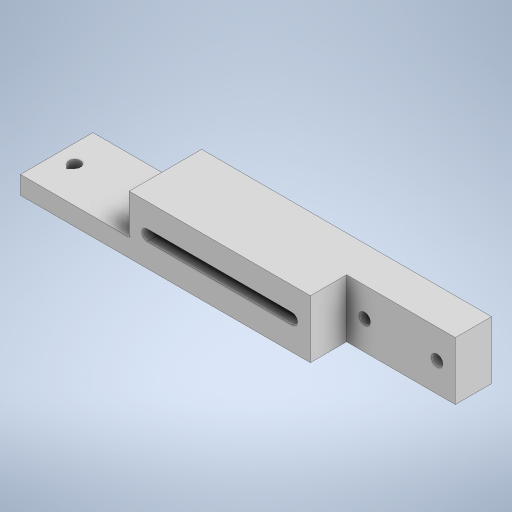
# Autodesk Inventor part: middle_hole
Saved by Autodesk Inventor 2023 (Build 270158000, 158)
## iProperties
Created: 2023-11-20
Part Number: middle_hole
Material: Všeobecné
Document SubType Name: Modeling
Designer: zavrel
Density: 1 g/cm^3
Appearance: Výchozí
Author: zavrel
Autodesk Inventor part; units mm, degrees
ref_plane "YZ Plane" through (0, 0, 0) normal (1, 0, 0) x (0, 1, 0)
ref_plane "XZ Plane" through (0, 0, 0) normal (0, 1, 0) x (-1, 0, 0)
ref_plane "XY Plane" through (0, 0, 0) normal (0, 0, 1) x (1, 0, 0)
sketch "Náčrt1" plane through (0, 0, 0) normal (0, 1, 0) x (-1, 0, 0)
  line L0 (0, 0) -> (110, 0)
  line L1 (110, 0) -> (110, -20)
  line L2 (110, -20) -> (0, -20)
  line L3 (0, -20) -> (0, 0)
  line L4 (55, -20) -> (55, 0) construction
  line L5 (110, -10) -> (0, -10) construction
  circle A0 centre (105, -10) radius 1.6
  circle A1 centre (85, -10) radius 1.6
  line L6 (105, -10) -> (105, -4.8731) construction
  line L7 (85, -10) -> (85, -4.8731) construction
  line L8 (105, -7.7373) -> (103.8686, -8.8686)
  line L9 (105, -7.7373) -> (106.1314, -8.8686)
  line L10 (85, -7.7373) -> (83.8686, -8.8686)
  line L11 (85, -7.7373) -> (86.1314, -8.8686)
  dimension "d0" = 20
  dimension "d1" = 110
  dimension "d4" = 3.2
  dimension "d6" = 25
  dimension "d7" = 5
  dimension "d49" = 90
  dimension "d50" = 90
  constraints: 24 end point, 4 midpoint, 3 point on line, 2 centre point, 2 parallel, 2 point on circle, 2 tangent, 2 vertical, 1 equal radius, 1 horizontal, 1 perpendicular
  measures "d0" distance between parallel lines of L2 L0
  measures "d1" distance of L1.end L2.end
  measures "d4" diameter of A0
  measures "d6" distance from line of L1 L7.start
  measures "d7" distance from line of L1 L6.start
  measures "d49" angle of L9 L8
  measures "d50" angle of L11 L10
extrude "Vysunutí1" add sketch "Náčrt1" along normal blind 16
sketch "Náčrt2" plane through (0, 16, 0) normal (0, 1, 0) x (1, 0, 0)
  line L0 (0, 20) -> (-110, 20) projected
  line L1 (-110, 20) -> (-110, 0) projected
  line L2 (-110, 0) -> (0, 0) projected
  line L3 (0, 0) -> (0, 20) projected
  arc A0 (-83.8686, 8.8686) -> (-86.1314, 8.8686) centre (-85, 10) ccw projected
  arc A1 (-103.8686, 8.8686) -> (-106.1314, 8.8686) centre (-105, 10) ccw projected
  line L4 (-80, 0) -> (-80, 20)
  line L5 (-30, 0) -> (-30, 20)
  arc A2 (-103.8686, 8.8686) -> (-106.1314, 8.8686) centre (-105, 10) ccw construction
  arc A3 (-83.8686, 8.8686) -> (-86.1314, 8.8686) centre (-85, 10) ccw projected
  line L6 (-85, 7.7373) -> (-86.1314, 8.8686) projected
  line L7 (-83.8686, 8.8686) -> (-85, 7.7373) projected
  line L8 (-105, 7.7373) -> (-106.1314, 8.8686) projected
  line L9 (-103.8686, 8.8686) -> (-105, 7.7373) projected
  point P0 (0, 10)
  point P1 (-30, 10)
  point P2 (-85, 7.7373)
  point P3 (-105, 7.7373)
  dimension "d10" = 30
  dimension "d11" = 30
  constraints: 4 end point, 4 point on line, 2 midpoint, 2 parallel
  measures "d10" distance between parallel lines of L1 L4
  measures "d11" distance of point (0, 10) point (-30, 10)
extrude "Vysunutí2" cut sketch "Náčrt2" against normal blind 11 contours L4 L2 L1 L0 | L7 L6 A0 | L9 L8 A1
sketch "Náčrt4" plane through (0, 0, 0) normal (0, -1, 0) x (1, 0, 0)
  line L0 (0, -20) -> (-110, -20) projected
  line L1 (0, 0) -> (0, -20) projected
  line L2 (-110, 0) -> (0, 0) projected
  line L3 (-110, -20) -> (-110, 0) projected
  arc A0 (-86.1314, -8.8686) -> (-83.8686, -8.8686) centre (-85, -10) ccw projected
  arc A1 (-106.1314, -8.8686) -> (-103.8686, -8.8686) centre (-105, -10) ccw projected
  arc A2 (-110, -20) -> (-110, -20) centre (-105, -10) ccw projected
  line L4 (-105, -6.8246) -> (-102.25, -8.4123)
  line L5 (-102.25, -8.4123) -> (-102.25, -11.5877)
  line L6 (-102.25, -11.5877) -> (-105, -13.1754)
  line L7 (-105, -13.1754) -> (-107.75, -11.5877)
  line L8 (-107.75, -11.5877) -> (-107.75, -8.4123)
  line L9 (-107.75, -8.4123) -> (-105, -6.8246)
  arc A3 (-110, -20) -> (-110, -20) centre (-85, -10) ccw projected
  line L10 (-84.9134, -6.8258) -> (-82.2077, -8.4879)
  line L11 (-82.2077, -8.4879) -> (-82.2943, -11.6621)
  line L12 (-82.2943, -11.6621) -> (-85.0866, -13.1742)
  line L13 (-85.0866, -13.1742) -> (-87.7923, -11.5121)
  line L14 (-87.7923, -11.5121) -> (-87.7057, -8.3379)
  line L15 (-87.7057, -8.3379) -> (-84.9134, -6.8258)
  line L16 (-85, -7.7373) -> (-86.1314, -8.8686) projected
  line L17 (-83.8686, -8.8686) -> (-85, -7.7373) projected
  line L18 (-105, -7.7373) -> (-106.1314, -8.8686) projected
  line L19 (-103.8686, -8.8686) -> (-105, -7.7373) projected
  point P0 (-102.25, -10)
  point P1 (-107.75, -10)
  dimension "d17" = 5.5
  constraints: 24 end point, 2 coincident, 2 midpoint, 1 equal length, 28 other
  measures "d17" distance of point (-102.25, -10) point (-107.75, -10)
extrude "Vysunutí4" cut sketch "Náčrt4" against normal blind 2.5 contours L16 L17 A0 | L18 L19 A1 | L4 L5 L6 L7 L8 L9 | L10 L11 L12 L13 L14 L15
sketch "Náčrt6" plane through (-110, 0, 0) normal (0, 0, 1) x (1, 0, 0)
  line L0 (0, 0) -> (0, 5) projected
  line L1 (0, 0) -> (110, 0) projected
  line L2 (110, 0) -> (110, 16) projected
  line L3 (30, 16) -> (110, 16) projected
  line L4 (110, 16) -> (0, 16) projected
  line L5 (80, 16) -> (80, 0)
  line L6 (30, 16) -> (30, 5) projected
  line L7 (30, 5) -> (0, 5) projected
  dimension "d24" = 30
  constraints: 2 end point, 2 point on line, 1 perpendicular
  measures "d24" distance between parallel lines of L2 L5
extrude "Vysunutí5" cut sketch "Náčrt6" against normal blind 10 contours L5 L3 L2 L1
sketch "Náčrt7" plane through (-110, 0, -10) normal (0, 0, 1) x (1, 0, 0)
  line L0 (80, 16) -> (110, 16) projected
  line L1 (80, 0) -> (80, 16) projected
  line L2 (110, 0) -> (80, 0) projected
  line L3 (110, 16) -> (110, 0) projected
  line L4 (110, 0) -> (110, 16) construction
  line L5 (110, 8) -> (80, 8) construction
  circle A0 centre (85, 8) radius 1.6
  circle A1 centre (105, 8) radius 1.6
  line L6 (85, 8) -> (85, 12.494) construction
  line L7 (105, 8) -> (105, 11.0554) construction
  line L8 (85, 10.2627) -> (83.8686, 9.1314)
  line L9 (85, 10.2627) -> (86.1314, 9.1314)
  line L10 (105, 10.2627) -> (103.8686, 9.1314)
  line L11 (105, 10.2627) -> (106.1314, 9.1314)
  dimension "d30" = 3.2
  dimension "d31" = 25
  dimension "d32" = 5
  dimension "d38" = 90
  dimension "d39" = 90
  constraints: 14 end point, 4 point on circle, 4 point on line, 4 tangent, 2 centre point, 2 midpoint, 2 vertical, 1 equal radius
  measures "d30" diameter of A0
  measures "d31" distance from line of L3 L6.start
  measures "d32" distance from line of L3 L7.start
  measures "d38" angle of L9 L8
  measures "d39" angle of L11 L10
extrude "Vysunutí6" cut sketch "Náčrt7" against normal through all contours A0 | A1
sketch "Náčrt8" plane through (0, 0, -20) normal (0, 0, -1) x (-1, 0, 0)
  circle A0 centre (5, 8) radius 1.6 projected
  circle A1 centre (25, 8) radius 1.6 projected
  line L0 (0, 16) -> (80, 16) projected
  line L1 (0, 0) -> (0, 16) projected
  line L2 (0, 0) -> (110, 0) projected
  line L3 (110, 0) -> (110, 5) projected
  line L4 (25, 4.8246) -> (22.25, 6.4123)
  line L5 (22.25, 6.4123) -> (22.25, 9.5877)
  line L6 (22.25, 9.5877) -> (25, 11.1754)
  line L7 (25, 11.1754) -> (27.75, 9.5877)
  line L8 (27.75, 9.5877) -> (27.75, 6.4123)
  line L9 (27.75, 6.4123) -> (25, 4.8246)
  line L10 (5, 4.8246) -> (2.25, 6.4123)
  line L11 (2.25, 6.4123) -> (2.25, 9.5877)
  line L12 (2.25, 9.5877) -> (5, 11.1754)
  line L13 (5, 11.1754) -> (7.75, 9.5877)
  line L14 (7.75, 9.5877) -> (7.75, 6.4123)
  line L15 (7.75, 6.4123) -> (5, 4.8246)
  line L16 (80, 5) -> (80, 16) projected
  line L17 (110, 5) -> (80, 5) projected
  dimension "d35" = 5.5
  constraints: 24 end point, 2 coincident, 1 parallel, 26 other
  measures "d35" distance between parallel lines of L5 L8
extrude "Vysunutí7" cut sketch "Náčrt8" against normal blind 2.5 contours A0 | A1 | L4 L5 L6 L7 L8 L9 | L10 L11 L12 L13 L14 L15
sketch "Náčrt10" plane through (-110, 5, 0) normal (0, 0, 1) x (1, 0, 0)
  line L0 (80, -5) -> (80, 11) projected
  line L1 (30, 11) -> (80, 11) projected
  line L2 (0, -5) -> (0, 0) projected
  line L3 (0, -5) -> (80, -5) projected
  circle A0 centre (105, 3) radius 1.6 projected
  circle A1 centre (85, 3) radius 1.6 projected
  line L4 (80, 11) -> (110, 11) projected
  line L5 (80, -5) -> (80, 11) projected
  line L6 (110, -5) -> (80, -5) projected
  line L7 (110, 11) -> (110, -5) projected
  line L8 (55, 22.3819) -> (55, -13.3022) construction
  line L9 (110, -5) -> (110, 11) construction
  line L10 (110, 3) -> (22.1304, 3) construction
  line L11 (35, 3) -> (75, 3) construction
  line L12 (35, 1.5) -> (75, 1.5)
  line L13 (75, 4.5) -> (35, 4.5)
  arc A2 (35, 4.5) -> (35, 1.5) centre (35, 3) ccw
  arc A3 (75, 1.5) -> (75, 4.5) centre (75, 3) ccw
  line L14 (110, -5) -> (0, -5) projected
  line L15 (30, 11) -> (30, 0) projected
  line L16 (30, 0) -> (0, 0) projected
  point P0 (55, 3)
  point P1 (55, -5)
  dimension "d43" = 3
  dimension "d44" = 40
  constraints: 12 end point, 4 point on circle, 4 point on line, 4 tangent, 3 midpoint, 2 centre point, 1 horizontal, 1 parallel, 1 vertical
  measures "d43" distance between parallel lines of L12 L13
  measures "d44" distance of L11.start L11.end
extrude "Vysunutí8" cut sketch "Náčrt10" against normal up to surface (20 mm away) contours A2 L13 A3 L12
